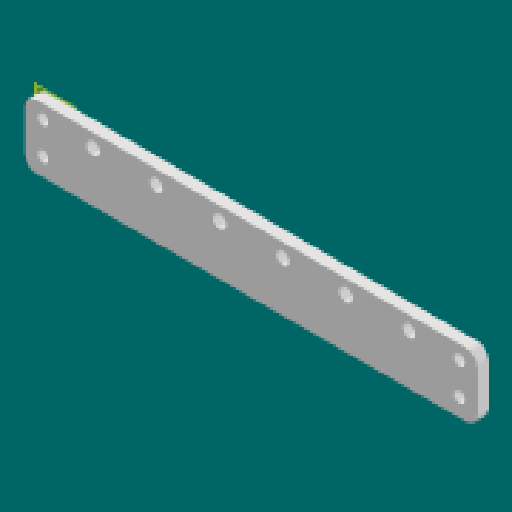
# Autodesk Inventor part: string_mount
Saved by Autodesk Inventor 2023 (Build 270158000, 158)
## iProperties
Created: 2022-11-12
Part Number: string_mount
Material: Generic
Document SubType Name: Modeling
Designer: sgodi
Density: 1 g/cm^3
Appearance: Default
Author: sgodi
Autodesk Inventor part; units mm, degrees
ref_plane "YZ Plane" through (0, 0, 0) normal (1, 0, 0) x (0, 1, 0)
ref_plane "XZ Plane" through (0, 0, 0) normal (0, 1, 0) x (-1, 0, 0)
ref_plane "XY Plane" through (0, 0, 0) normal (0, 0, 1) x (1, 0, 0)
ref_plane "Work Plane2" through (0, 147.11, 157.65) normal (0, 0, 1) x (1, 0, 0)
sketch "Sketch2" plane through (0, 147.11, 157.65) normal (0, 0, 1) x (1, 0, 0)
  arc A0 (61.9417, -3.175) -> (58.7667, 0) centre (58.7667, -3.175) ccw projected
  line L0 (58.7667, 0) -> (55.1167, 0) projected
  arc A1 (51.9417, 3.175) -> (55.1167, 0) centre (55.1167, 3.175) ccw projected
  arc A2 (51.9417, 3.937) -> (48.7667, 7.112) centre (48.7667, 3.937) ccw projected
  line L1 (48.7667, 7.112) -> (-48.7667, 7.112) projected
  arc A3 (-48.7667, 7.112) -> (-51.9417, 3.937) centre (-48.7667, 3.937) ccw projected
  arc A4 (-55.1167, 0) -> (-51.9417, 3.175) centre (-55.1167, 3.175) ccw projected
  line L2 (-55.1167, 0) -> (-58.7667, 0) projected
  arc A5 (-58.7667, 0) -> (-61.9417, -3.175) centre (-58.7667, -3.175) ccw projected
  line L3 (-61.9417, -3.175) -> (-61.9417, -14.325) projected
  arc A6 (-61.9417, -14.325) -> (-58.7667, -17.5) centre (-58.7667, -14.325) ccw projected
  line L4 (-58.7667, -17.5) -> (58.7667, -17.5) projected
  arc A7 (58.7667, -17.5) -> (61.9417, -14.325) centre (58.7667, -14.325) ccw projected
  line L5 (61.9417, -14.325) -> (61.9417, -3.175) projected
  arc A8 (-44.4178, 0) -> (-42.1518, 0) centre (-43.2848, 0) ccw projected
  line L6 (-44.4178, 0) -> (-44.4178, 5) projected
  arc A9 (-42.1518, 5) -> (-44.4178, 5) centre (-43.2848, 5) ccw projected
  line L7 (-42.1518, 5) -> (-42.1518, 0) projected
  circle A10 centre (56.9417, -12.5) radius 1.524 projected
  circle A11 centre (-56.9417, -3.75) radius 1.524 projected
  circle A12 centre (56.9417, -3.75) radius 1.524 projected
  circle A13 centre (-43.2848, -3.75) radius 1.27 projected
  circle A14 centre (-25.9709, -3.75) radius 1.27 projected
  circle A15 centre (-8.657, -3.75) radius 1.27 projected
  circle A16 centre (8.657, -3.75) radius 1.27 projected
  circle A17 centre (25.9709, -3.75) radius 1.27 projected
  circle A18 centre (43.2848, -3.75) radius 1.27 projected
  circle A19 centre (-56.9417, -12.5) radius 1.524 projected
  arc A20 (-27.1039, 0) -> (-24.8379, 0) centre (-25.9709, 0) ccw projected
  line L8 (-27.1039, 0) -> (-27.1039, 5) projected
  arc A21 (-24.8379, 5) -> (-27.1039, 5) centre (-25.9709, 5) ccw projected
  line L9 (-24.8379, 5) -> (-24.8379, 0) projected
  arc A22 (-9.79, 0) -> (-7.524, 0) centre (-8.657, 0) ccw projected
  line L10 (-9.79, 0) -> (-9.79, 5) projected
  arc A23 (-7.524, 5) -> (-9.79, 5) centre (-8.657, 5) ccw projected
  line L11 (-7.524, 5) -> (-7.524, 0) projected
  arc A24 (7.524, 0) -> (9.79, 0) centre (8.657, 0) ccw projected
  line L12 (7.524, 0) -> (7.524, 5) projected
  arc A25 (9.79, 5) -> (7.524, 5) centre (8.657, 5) ccw projected
  line L13 (9.79, 5) -> (9.79, 0) projected
  arc A26 (24.8379, 0) -> (27.1039, 0) centre (25.9709, 0) ccw projected
  line L14 (24.8379, 0) -> (24.8379, 5) projected
  arc A27 (27.1039, 5) -> (24.8379, 5) centre (25.9709, 5) ccw projected
  line L15 (27.1039, 5) -> (27.1039, 0) projected
  arc A28 (42.1518, 0) -> (44.4178, 0) centre (43.2848, 0) ccw projected
  line L16 (42.1518, 0) -> (42.1518, 5) projected
  arc A29 (44.4178, 5) -> (42.1518, 5) centre (43.2848, 5) ccw projected
  line L17 (44.4178, 5) -> (44.4178, 0) projected
  line L18 (-55.1167, 0) -> (55.1167, 0)
  circle A30 centre (-43.2848, -3.75) radius 1.778
  circle A31 centre (-25.9709, -3.75) radius 1.778
  circle A32 centre (-8.657, -3.75) radius 1.778
  circle A33 centre (8.657, -3.75) radius 1.778
  circle A34 centre (25.9709, -3.75) radius 1.778
  circle A35 centre (43.2848, -3.75) radius 1.778
  line L19 (-54.3979, -17.5) -> (54.3979, -17.5)
  line L20 (51.9417, 3.175) -> (51.9417, 3.937) projected
  line L21 (-51.9417, 3.937) -> (-51.9417, 3.175) projected
  point P0 (0, -147.11)
  point P1 (-55.1167, 3.175)
  point P2 (51.9417, 3.683)
  point P3 (-51.9417, 3.683)
  point P4 (-55.1167, 3.175)
  dimension "d0" = 3.556
  dimension "d1" = 3.556
  dimension "d2" = 3.556
  dimension "d3" = 3.556
  dimension "d4" = 3.556
  dimension "d5" = 3.556
  constraints: 6 centre point, 6 coincident, 4 end point, 1 collinear, 1 horizontal, 1 tangent
  measures "d0" diameter of A30
  measures "d1" diameter of A31
  measures "d2" diameter of A32
  measures "d3" diameter of A33
  measures "d4" diameter of A34
  measures "d5" diameter of A35
extrude "Extrusion1" add sketch "Sketch2" along normal blind 3.175 contours L5 A7 L4 A6 L3 A5 L2 L18 A8 A20 A22 A24 A26 A28 L0 A0 | A28 L18 | A26 L18 | A24 L18 | A22 L18 | L18 A8 | A20 L18
body "Solid1"
